Autodesk Fusion 360 part; units mm, degrees
(part 11 of 40)
  line L4767 (177.1415, 206.1712) -> (177.0096, 206.2642) construction
  line L4768 (177.0096, 206.2642) -> (176.8768, 206.3564) construction
  line L4769 (176.8768, 206.3564) -> (176.7434, 206.448) construction
  line L4770 (176.7434, 206.448) -> (176.6092, 206.5388) construction
  line L4771 (176.6092, 206.5388) -> (176.4743, 206.629) construction
  line L4772 (176.4743, 206.629) -> (176.3387, 206.7185) construction
  line L4773 (176.3387, 206.7185) -> (176.2025, 206.8073) construction
  line L4774 (176.2025, 206.8073) -> (176.0655, 206.8955) construction
  line L4775 (176.0655, 206.8955) -> (175.9278, 206.9829) construction
  line L4776 (175.9278, 206.9829) -> (175.7895, 207.0697) construction
  line L4777 (175.7895, 207.0697) -> (175.6505, 207.1558) construction
  line L4778 (175.6505, 207.1558) -> (175.5109, 207.2413) construction
  line L4779 (175.5109, 207.2413) -> (175.3706, 207.3261) construction
  line L4780 (175.3706, 207.3261) -> (175.2297, 207.4102) construction
  line L4781 (175.2297, 207.4102) -> (175.0882, 207.4937) construction
  line L4782 (175.0882, 207.4937) -> (174.946, 207.5765) construction
  line L4783 (174.946, 207.5765) -> (174.8032, 207.6587) construction
  line L4784 (174.8032, 207.6587) -> (174.6599, 207.7403) construction
  line L4785 (174.6599, 207.7403) -> (174.5159, 207.8212) construction
  line L4786 (174.5159, 207.8212) -> (174.3713, 207.9014) construction
  line L4787 (174.3713, 207.9014) -> (174.2262, 207.981) construction
  line L4788 (174.2262, 207.981) -> (174.0805, 208.06) construction
  line L4789 (174.0805, 208.06) -> (173.9342, 208.1383) construction
  line L4790 (173.9342, 208.1383) -> (173.7873, 208.216) construction
  line L4791 (173.7873, 208.216) -> (173.6399, 208.2931) construction
  line L4792 (173.6399, 208.2931) -> (173.4919, 208.3695) construction
  line L4793 (173.4919, 208.3695) -> (173.3434, 208.4453) construction
  line L4794 (173.3434, 208.4453) -> (173.1943, 208.5205) construction
  line L4795 (173.1943, 208.5205) -> (173.0447, 208.595) construction
  line L4796 (173.0447, 208.595) -> (172.8946, 208.669) construction
  line L4797 (172.8946, 208.669) -> (172.7439, 208.7423) construction
  line L4798 (172.7439, 208.7423) -> (172.5927, 208.8149) construction
  line L4799 (172.5927, 208.8149) -> (172.4411, 208.887) construction
  line L4800 (172.4411, 208.887) -> (172.2889, 208.9584) construction
  line L4801 (172.2889, 208.9584) -> (172.1667, 209.0151) construction
  line L4802 (172.1667, 209.0151) -> (172.0748, 209.0573) construction
  line L4803 (172.0748, 209.0573) -> (172.0135, 209.0853) construction
  line L4804 (172.0135, 209.0853) -> (171.9828, 209.0993) construction
  arc A128 (279.3511, 125.7868) -> (280.7456, 130.0785) centre (212.132, 150) ccw
  arc A129 (171.9828, 209.0993) -> (168.332, 206.4469) centre (212.132, 150) ccw
  spline S64 degree 5 poles (217.8271, 210.7685) (217.8299, 210.7993) (217.8349, 210.8609) (217.8398, 210.9533) (217.8417, 211.0766) (217.8376, 211.231) (217.8289, 211.3856) (217.8174, 211.5403) (217.8043, 211.695) (217.7903, 211.8498) (217.7751, 212.0045) (217.7585, 212.1593) (217.74, 212.314) (217.7191, 212.4688) (217.6961, 212.6235) (217.671, 212.7782) (217.6441, 212.9329) (217.6158, 213.0875) (217.5862, 213.2421) (217.5553, 213.3966) (217.5233, 213.5511) (217.4899, 213.7055) (217.4552, 213.8598) (217.4191, 214.014) (217.3817, 214.1682) (217.3429, 214.3222) (217.3029, 214.4762) (217.2617, 214.6301) (217.2193, 214.7839) (217.1759, 214.9376) (217.1313, 215.0912) (217.0856, 215.2447) (217.0388, 215.398) (216.9909, 215.5513) (216.9419, 215.7044) (216.8919, 215.8574) (216.8407, 216.0103) (216.7886, 216.1631) (216.7355, 216.3158) (216.6813, 216.4683) (216.6262, 216.6206) (216.57, 216.7729) (216.513, 216.925) (216.4549, 217.077) (216.3959, 217.2288) (216.3359, 217.3804) (216.275, 217.532) (216.2132, 217.6833) (216.1505, 217.8345) (216.0868, 217.9856) (216.0223, 218.1365) (215.9569, 218.2872) (215.8905, 218.4378) (215.8233, 218.5882) (215.7553, 218.7384) (215.6863, 218.8885) (215.6166, 219.0384) (215.5459, 219.1881) (215.4745, 219.3376) (215.4021, 219.487) (215.329, 219.6362) (215.255, 219.7852) (215.1802, 219.934) (215.1046, 220.0826) (215.0282, 220.2311) (214.951, 220.3793) (214.873, 220.5274) (214.7942, 220.6752) (214.7146, 220.8229) (214.6343, 220.9703) (214.5531, 221.1176) (214.4876, 221.2352) (214.4381, 221.3234) (214.4049, 221.3821) (214.3883, 221.4115) knots 0 0 0 0 0 0 0.01428571 0.02857143 0.04285714 0.05714286 0.07142857 0.08571429 0.1 0.11428571 0.12857143 0.14285714 0.15714286 0.17142857 0.18571429 0.2 0.21428571 0.22857143 0.24285714 0.25714286 0.27142857 0.28571429 0.3 0.31428571 0.32857143 0.34285714 0.35714286 0.37142857 0.38571429 0.4 0.41428571 0.42857143 0.44285714 0.45714286 0.47142857 0.48571429 0.5 0.51428571 0.52857143 0.54285714 0.55714286 0.57142857 0.58571429 0.6 0.61428571 0.62857143 0.64285714 0.65714286 0.67142857 0.68571429 0.7 0.71428571 0.72857143 0.74285714 0.75714286 0.77142857 0.78571429 0.8 0.81428571 0.82857143 0.84285714 0.85714286 0.87142857 0.88571429 0.9 0.91428571 0.92857143 0.94285714 0.95714286 0.97142857 0.98571429 1 1 1 1 1 1
  line L4805 (217.8271, 210.7685) -> (217.8299, 210.7993) construction
  line L4806 (217.8299, 210.7993) -> (217.8349, 210.8609) construction
  line L4807 (217.8349, 210.8609) -> (217.8398, 210.9533) construction
  line L4808 (217.8398, 210.9533) -> (217.8417, 211.0766) construction
  line L4809 (217.8417, 211.0766) -> (217.8376, 211.231) construction
  line L4810 (217.8376, 211.231) -> (217.8289, 211.3856) construction
  line L4811 (217.8289, 211.3856) -> (217.8174, 211.5403) construction
  line L4812 (217.8174, 211.5403) -> (217.8043, 211.695) construction
  line L4813 (217.8043, 211.695) -> (217.7903, 211.8498) construction
  line L4814 (217.7903, 211.8498) -> (217.7751, 212.0045) construction
  line L4815 (217.7751, 212.0045) -> (217.7585, 212.1593) construction
  line L4816 (217.7585, 212.1593) -> (217.74, 212.314) construction
  line L4817 (217.74, 212.314) -> (217.7191, 212.4688) construction
  line L4818 (217.7191, 212.4688) -> (217.6961, 212.6235) construction
  line L4819 (217.6961, 212.6235) -> (217.671, 212.7782) construction
  line L4820 (217.671, 212.7782) -> (217.6441, 212.9329) construction
  line L4821 (217.6441, 212.9329) -> (217.6158, 213.0875) construction
  line L4822 (217.6158, 213.0875) -> (217.5862, 213.2421) construction
  line L4823 (217.5862, 213.2421) -> (217.5553, 213.3966) construction
  line L4824 (217.5553, 213.3966) -> (217.5233, 213.5511) construction
  line L4825 (217.5233, 213.5511) -> (217.4899, 213.7055) construction
  line L4826 (217.4899, 213.7055) -> (217.4552, 213.8598) construction
  line L4827 (217.4552, 213.8598) -> (217.4191, 214.014) construction
  line L4828 (217.4191, 214.014) -> (217.3817, 214.1682) construction
  line L4829 (217.3817, 214.1682) -> (217.3429, 214.3222) construction
  line L4830 (217.3429, 214.3222) -> (217.3029, 214.4762) construction
  line L4831 (217.3029, 214.4762) -> (217.2617, 214.6301) construction
  line L4832 (217.2617, 214.6301) -> (217.2193, 214.7839) construction
  line L4833 (217.2193, 214.7839) -> (217.1759, 214.9376) construction
  line L4834 (217.1759, 214.9376) -> (217.1313, 215.0912) construction
  line L4835 (217.1313, 215.0912) -> (217.0856, 215.2447) construction
  line L4836 (217.0856, 215.2447) -> (217.0388, 215.398) construction
  line L4837 (217.0388, 215.398) -> (216.9909, 215.5513) construction
  line L4838 (216.9909, 215.5513) -> (216.9419, 215.7044) construction
  line L4839 (216.9419, 215.7044) -> (216.8919, 215.8574) construction
  line L4840 (216.8919, 215.8574) -> (216.8407, 216.0103) construction
  line L4841 (216.8407, 216.0103) -> (216.7886, 216.1631) construction
  line L4842 (216.7886, 216.1631) -> (216.7355, 216.3158) construction
  line L4843 (216.7355, 216.3158) -> (216.6813, 216.4683) construction
  line L4844 (216.6813, 216.4683) -> (216.6262, 216.6206) construction
  line L4845 (216.6262, 216.6206) -> (216.57, 216.7729) construction
  line L4846 (216.57, 216.7729) -> (216.513, 216.925) construction
  line L4847 (216.513, 216.925) -> (216.4549, 217.077) construction
  line L4848 (216.4549, 217.077) -> (216.3959, 217.2288) construction
  line L4849 (216.3959, 217.2288) -> (216.3359, 217.3804) construction
  line L4850 (216.3359, 217.3804) -> (216.275, 217.532) construction
  line L4851 (216.275, 217.532) -> (216.2132, 217.6833) construction
  line L4852 (216.2132, 217.6833) -> (216.1505, 217.8345) construction
  line L4853 (216.1505, 217.8345) -> (216.0868, 217.9856) construction
  line L4854 (216.0868, 217.9856) -> (216.0223, 218.1365) construction
  line L4855 (216.0223, 218.1365) -> (215.9569, 218.2872) construction
  line L4856 (215.9569, 218.2872) -> (215.8905, 218.4378) construction
  line L4857 (215.8905, 218.4378) -> (215.8233, 218.5882) construction
  line L4858 (215.8233, 218.5882) -> (215.7553, 218.7384) construction
  line L4859 (215.7553, 218.7384) -> (215.6863, 218.8885) construction
  line L4860 (215.6863, 218.8885) -> (215.6166, 219.0384) construction
  line L4861 (215.6166, 219.0384) -> (215.5459, 219.1881) construction
  line L4862 (215.5459, 219.1881) -> (215.4745, 219.3376) construction
  line L4863 (215.4745, 219.3376) -> (215.4021, 219.487) construction
  line L4864 (215.4021, 219.487) -> (215.329, 219.6362) construction
  line L4865 (215.329, 219.6362) -> (215.255, 219.7852) construction
  line L4866 (215.255, 219.7852) -> (215.1802, 219.934) construction
  line L4867 (215.1802, 219.934) -> (215.1046, 220.0826) construction
  line L4868 (215.1046, 220.0826) -> (215.0282, 220.2311) construction
  line L4869 (215.0282, 220.2311) -> (214.951, 220.3793) construction
  line L4870 (214.951, 220.3793) -> (214.873, 220.5274) construction
  line L4871 (214.873, 220.5274) -> (214.7942, 220.6752) construction
  line L4872 (214.7942, 220.6752) -> (214.7146, 220.8229) construction
  line L4873 (214.7146, 220.8229) -> (214.6343, 220.9703) construction
  line L4874 (214.6343, 220.9703) -> (214.5531, 221.1176) construction
  line L4875 (214.5531, 221.1176) -> (214.4876, 221.2352) construction
  line L4876 (214.4876, 221.2352) -> (214.4381, 221.3234) construction
  line L4877 (214.4381, 221.3234) -> (214.4049, 221.3821) construction
  line L4878 (214.4049, 221.3821) -> (214.3883, 221.4115) construction
  arc A130 (171.9828, 209.0993) -> (168.332, 206.4469) centre (212.132, 150) ccw
  spline S65 degree 5 poles (217.8271, 210.7685) (217.8299, 210.7993) (217.8349, 210.8609) (217.8398, 210.9533) (217.8417, 211.0766) (217.8376, 211.231) (217.8289, 211.3856) (217.8174, 211.5403) (217.8043, 211.695) (217.7903, 211.8498) (217.7751, 212.0045) (217.7585, 212.1593) (217.74, 212.314) (217.7191, 212.4688) (217.6961, 212.6235) (217.671, 212.7782) (217.6441, 212.9329) (217.6158, 213.0875) (217.5862, 213.2421) (217.5553, 213.3966) (217.5233, 213.5511) (217.4899, 213.7055) (217.4552, 213.8598) (217.4191, 214.014) (217.3817, 214.1682) (217.3429, 214.3222) (217.3029, 214.4762) (217.2617, 214.6301) (217.2193, 214.7839) (217.1759, 214.9376) (217.1313, 215.0912) (217.0856, 215.2447) (217.0388, 215.398) (216.9909, 215.5513) (216.9419, 215.7044) (216.8919, 215.8574) (216.8407, 216.0103) (216.7886, 216.1631) (216.7355, 216.3158) (216.6813, 216.4683) (216.6262, 216.6206) (216.57, 216.7729) (216.513, 216.925) (216.4549, 217.077) (216.3959, 217.2288) (216.3359, 217.3804) (216.275, 217.532) (216.2132, 217.6833) (216.1505, 217.8345) (216.0868, 217.9856) (216.0223, 218.1365) (215.9569, 218.2872) (215.8905, 218.4378) (215.8233, 218.5882) (215.7553, 218.7384) (215.6863, 218.8885) (215.6166, 219.0384) (215.5459, 219.1881) (215.4745, 219.3376) (215.4021, 219.487) (215.329, 219.6362) (215.255, 219.7852) (215.1802, 219.934) (215.1046, 220.0826) (215.0282, 220.2311) (214.951, 220.3793) (214.873, 220.5274) (214.7942, 220.6752) (214.7146, 220.8229) (214.6343, 220.9703) (214.5531, 221.1176) (214.4876, 221.2352) (214.4381, 221.3234) (214.4049, 221.3821) (214.3883, 221.4115) knots 0 0 0 0 0 0 0.01428571 0.02857143 0.04285714 0.05714286 0.07142857 0.08571429 0.1 0.11428571 0.12857143 0.14285714 0.15714286 0.17142857 0.18571429 0.2 0.21428571 0.22857143 0.24285714 0.25714286 0.27142857 0.28571429 0.3 0.31428571 0.32857143 0.34285714 0.35714286 0.37142857 0.38571429 0.4 0.41428571 0.42857143 0.44285714 0.45714286 0.47142857 0.48571429 0.5 0.51428571 0.52857143 0.54285714 0.55714286 0.57142857 0.58571429 0.6 0.61428571 0.62857143 0.64285714 0.65714286 0.67142857 0.68571429 0.7 0.71428571 0.72857143 0.74285714 0.75714286 0.77142857 0.78571429 0.8 0.81428571 0.82857143 0.84285714 0.85714286 0.87142857 0.88571429 0.9 0.91428571 0.92857143 0.94285714 0.95714286 0.97142857 0.98571429 1 1 1 1 1 1
  line L4879 (217.8271, 210.7685) -> (217.8299, 210.7993) construction
  line L4880 (217.8299, 210.7993) -> (217.8349, 210.8609) construction
  line L4881 (217.8349, 210.8609) -> (217.8398, 210.9533) construction
  line L4882 (217.8398, 210.9533) -> (217.8417, 211.0766) construction
  line L4883 (217.8417, 211.0766) -> (217.8376, 211.231) construction
  line L4884 (217.8376, 211.231) -> (217.8289, 211.3856) construction
  line L4885 (217.8289, 211.3856) -> (217.8174, 211.5403) construction
  line L4886 (217.8174, 211.5403) -> (217.8043, 211.695) construction
  line L4887 (217.8043, 211.695) -> (217.7903, 211.8498) construction
  line L4888 (217.7903, 211.8498) -> (217.7751, 212.0045) construction
  line L4889 (217.7751, 212.0045) -> (217.7585, 212.1593) construction
  line L4890 (217.7585, 212.1593) -> (217.74, 212.314) construction
  line L4891 (217.74, 212.314) -> (217.7191, 212.4688) construction
  line L4892 (217.7191, 212.4688) -> (217.6961, 212.6235) construction
  line L4893 (217.6961, 212.6235) -> (217.671, 212.7782) construction
  line L4894 (217.671, 212.7782) -> (217.6441, 212.9329) construction
  line L4895 (217.6441, 212.9329) -> (217.6158, 213.0875) construction
  line L4896 (217.6158, 213.0875) -> (217.5862, 213.2421) construction
  line L4897 (217.5862, 213.2421) -> (217.5553, 213.3966) construction
  line L4898 (217.5553, 213.3966) -> (217.5233, 213.5511) construction
  line L4899 (217.5233, 213.5511) -> (217.4899, 213.7055) construction
  line L4900 (217.4899, 213.7055) -> (217.4552, 213.8598) construction
  line L4901 (217.4552, 213.8598) -> (217.4191, 214.014) construction
  line L4902 (217.4191, 214.014) -> (217.3817, 214.1682) construction
  line L4903 (217.3817, 214.1682) -> (217.3429, 214.3222) construction
  line L4904 (217.3429, 214.3222) -> (217.3029, 214.4762) construction
  line L4905 (217.3029, 214.4762) -> (217.2617, 214.6301) construction
  line L4906 (217.2617, 214.6301) -> (217.2193, 214.7839) construction
  line L4907 (217.2193, 214.7839) -> (217.1759, 214.9376) construction
  line L4908 (217.1759, 214.9376) -> (217.1313, 215.0912) construction
  line L4909 (217.1313, 215.0912) -> (217.0856, 215.2447) construction
  line L4910 (217.0856, 215.2447) -> (217.0388, 215.398) construction
  line L4911 (217.0388, 215.398) -> (216.9909, 215.5513) construction
  line L4912 (216.9909, 215.5513) -> (216.9419, 215.7044) construction
  line L4913 (216.9419, 215.7044) -> (216.8919, 215.8574) construction
  line L4914 (216.8919, 215.8574) -> (216.8407, 216.0103) construction
  line L4915 (216.8407, 216.0103) -> (216.7886, 216.1631) construction
  line L4916 (216.7886, 216.1631) -> (216.7355, 216.3158) construction
  line L4917 (216.7355, 216.3158) -> (216.6813, 216.4683) construction
  line L4918 (216.6813, 216.4683) -> (216.6262, 216.6206) construction
  line L4919 (216.6262, 216.6206) -> (216.57, 216.7729) construction
  line L4920 (216.57, 216.7729) -> (216.513, 216.925) construction
  line L4921 (216.513, 216.925) -> (216.4549, 217.077) construction
  line L4922 (216.4549, 217.077) -> (216.3959, 217.2288) construction
  line L4923 (216.3959, 217.2288) -> (216.3359, 217.3804) construction
  line L4924 (216.3359, 217.3804) -> (216.275, 217.532) construction
  line L4925 (216.275, 217.532) -> (216.2132, 217.6833) construction
  line L4926 (216.2132, 217.6833) -> (216.1505, 217.8345) construction
  line L4927 (216.1505, 217.8345) -> (216.0868, 217.9856) construction
  line L4928 (216.0868, 217.9856) -> (216.0223, 218.1365) construction
  line L4929 (216.0223, 218.1365) -> (215.9569, 218.2872) construction
  line L4930 (215.9569, 218.2872) -> (215.8905, 218.4378) construction
  line L4931 (215.8905, 218.4378) -> (215.8233, 218.5882) construction
  line L4932 (215.8233, 218.5882) -> (215.7553, 218.7384) construction
  line L4933 (215.7553, 218.7384) -> (215.6863, 218.8885) construction
  line L4934 (215.6863, 218.8885) -> (215.6166, 219.0384) construction
  line L4935 (215.6166, 219.0384) -> (215.5459, 219.1881) construction
  line L4936 (215.5459, 219.1881) -> (215.4745, 219.3376) construction
  line L4937 (215.4745, 219.3376) -> (215.4021, 219.487) construction
  line L4938 (215.4021, 219.487) -> (215.329, 219.6362) construction
  line L4939 (215.329, 219.6362) -> (215.255, 219.7852) construction
  line L4940 (215.255, 219.7852) -> (215.1802, 219.934) construction
  line L4941 (215.1802, 219.934) -> (215.1046, 220.0826) construction
  line L4942 (215.1046, 220.0826) -> (215.0282, 220.2311) construction
  line L4943 (215.0282, 220.2311) -> (214.951, 220.3793) construction
  line L4944 (214.951, 220.3793) -> (214.873, 220.5274) construction
  line L4945 (214.873, 220.5274) -> (214.7942, 220.6752) construction
  line L4946 (214.7942, 220.6752) -> (214.7146, 220.8229) construction
  line L4947 (214.7146, 220.8229) -> (214.6343, 220.9703) construction
  line L4948 (214.6343, 220.9703) -> (214.5531, 221.1176) construction
  line L4949 (214.5531, 221.1176) -> (214.4876, 221.2352) construction
  line L4950 (214.4876, 221.2352) -> (214.4381, 221.3234) construction
  line L4951 (214.4381, 221.3234) -> (214.4049, 221.3821) construction
  line L4952 (214.4049, 221.3821) -> (214.3883, 221.4115) construction
  spline S66 degree 5 poles (206.4369, 210.7685) (206.4341, 210.7993) (206.4291, 210.8609) (206.4242, 210.9533) (206.4223, 211.0766) (206.4264, 211.231) (206.4351, 211.3856) (206.4466, 211.5403) (206.4597, 211.695) (206.4737, 211.8498) (206.4889, 212.0045) (206.5055, 212.1593) (206.524, 212.314) (206.5449, 212.4688) (206.5679, 212.6235) (206.593, 212.7782) (206.6199, 212.9329) (206.6482, 213.0875) (206.6778, 213.2421) (206.7087, 213.3966) (206.7407, 213.5511) (206.7741, 213.7055) (206.8088, 213.8598) (206.8449, 214.014) (206.8823, 214.1682) (206.9211, 214.3222) (206.9611, 214.4762) (207.0023, 214.6301) (207.0447, 214.7839) (207.0881, 214.9376) (207.1327, 215.0912) (207.1784, 215.2447) (207.2252, 215.398) (207.2731, 215.5513) (207.3221, 215.7044) (207.3721, 215.8574) (207.4233, 216.0103) (207.4754, 216.1631) (207.5285, 216.3158) (207.5827, 216.4683) (207.6378, 216.6206) (207.694, 216.7729) (207.751, 216.925) (207.8091, 217.077) (207.8681, 217.2288) (207.9281, 217.3804) (207.989, 217.532) (208.0508, 217.6833) (208.1135, 217.8345) (208.1772, 217.9856) (208.2417, 218.1365) (208.3071, 218.2872) (208.3735, 218.4378) (208.4407, 218.5882) (208.5087, 218.7384) (208.5777, 218.8885) (208.6474, 219.0384) (208.7181, 219.1881) (208.7895, 219.3376) (208.8619, 219.487) (208.935, 219.6362) (209.009, 219.7852) (209.0838, 219.934) (209.1594, 220.0826) (209.2358, 220.2311) (209.313, 220.3793) (209.391, 220.5274) (209.4698, 220.6752) (209.5494, 220.8229) (209.6297, 220.9703) (209.7109, 221.1176) (209.7764, 221.2352) (209.8259, 221.3234) (209.8591, 221.3821) (209.8757, 221.4115) knots 0 0 0 0 0 0 0.01428571 0.02857143 0.04285714 0.05714286 0.07142857 0.08571429 0.1 0.11428571 0.12857143 0.14285714 0.15714286 0.17142857 0.18571429 0.2 0.21428571 0.22857143 0.24285714 0.25714286 0.27142857 0.28571429 0.3 0.31428571 0.32857143 0.34285714 0.35714286 0.37142857 0.38571429 0.4 0.41428571 0.42857143 0.44285714 0.45714286 0.47142857 0.48571429 0.5 0.51428571 0.52857143 0.54285714 0.55714286 0.57142857 0.58571429 0.6 0.61428571 0.62857143 0.64285714 0.65714286 0.67142857 0.68571429 0.7 0.71428571 0.72857143 0.74285714 0.75714286 0.77142857 0.78571429 0.8 0.81428571 0.82857143 0.84285714 0.85714286 0.87142857 0.88571429 0.9 0.91428571 0.92857143 0.94285714 0.95714286 0.97142857 0.98571429 1 1 1 1 1 1
  line L4953 (206.4369, 210.7685) -> (206.4341, 210.7993) construction
  line L4954 (206.4341, 210.7993) -> (206.4291, 210.8609) construction
  line L4955 (206.4291, 210.8609) -> (206.4242, 210.9533) construction
  line L4956 (206.4242, 210.9533) -> (206.4223, 211.0766) construction
  line L4957 (206.4223, 211.0766) -> (206.4264, 211.231) construction
  line L4958 (206.4264, 211.231) -> (206.4351, 211.3856) construction
  line L4959 (206.4351, 211.3856) -> (206.4466, 211.5403) construction
  line L4960 (206.4466, 211.5403) -> (206.4597, 211.695) construction
  line L4961 (206.4597, 211.695) -> (206.4737, 211.8498) construction
  line L4962 (206.4737, 211.8498) -> (206.4889, 212.0045) construction
  line L4963 (206.4889, 212.0045) -> (206.5055, 212.1593) construction
  line L4964 (206.5055, 212.1593) -> (206.524, 212.314) construction
  line L4965 (206.524, 212.314) -> (206.5449, 212.4688) construction
  line L4966 (206.5449, 212.4688) -> (206.5679, 212.6235) construction
  line L4967 (206.5679, 212.6235) -> (206.593, 212.7782) construction
  line L4968 (206.593, 212.7782) -> (206.6199, 212.9329) construction
  line L4969 (206.6199, 212.9329) -> (206.6482, 213.0875) construction
  line L4970 (206.6482, 213.0875) -> (206.6778, 213.2421) construction
  line L4971 (206.6778, 213.2421) -> (206.7087, 213.3966) construction
  line L4972 (206.7087, 213.3966) -> (206.7407, 213.5511) construction
  line L4973 (206.7407, 213.5511) -> (206.7741, 213.7055) construction
  line L4974 (206.7741, 213.7055) -> (206.8088, 213.8598) construction
  line L4975 (206.8088, 213.8598) -> (206.8449, 214.014) construction
  line L4976 (206.8449, 214.014) -> (206.8823, 214.1682) construction
  line L4977 (206.8823, 214.1682) -> (206.9211, 214.3222) construction
  line L4978 (206.9211, 214.3222) -> (206.9611, 214.4762) construction
  line L4979 (206.9611, 214.4762) -> (207.0023, 214.6301) construction
  line L4980 (207.0023, 214.6301) -> (207.0447, 214.7839) construction
  line L4981 (207.0447, 214.7839) -> (207.0881, 214.9376) construction
  line L4982 (207.0881, 214.9376) -> (207.1327, 215.0912) construction
  line L4983 (207.1327, 215.0912) -> (207.1784, 215.2447) construction
  line L4984 (207.1784, 215.2447) -> (207.2252, 215.398) construction
  line L4985 (207.2252, 215.398) -> (207.2731, 215.5513) construction
  line L4986 (207.2731, 215.5513) -> (207.3221, 215.7044) construction
  line L4987 (207.3221, 215.7044) -> (207.3721, 215.8574) construction
  line L4988 (207.3721, 215.8574) -> (207.4233, 216.0103) construction
  line L4989 (207.4233, 216.0103) -> (207.4754, 216.1631) construction
  line L4990 (207.4754, 216.1631) -> (207.5285, 216.3158) construction
  line L4991 (207.5285, 216.3158) -> (207.5827, 216.4683) construction
  line L4992 (207.5827, 216.4683) -> (207.6378, 216.6206) construction
  line L4993 (207.6378, 216.6206) -> (207.694, 216.7729) construction
  line L4994 (207.694, 216.7729) -> (207.751, 216.925) construction
  line L4995 (207.751, 216.925) -> (207.8091, 217.077) construction
  line L4996 (207.8091, 217.077) -> (207.8681, 217.2288) construction
  line L4997 (207.8681, 217.2288) -> (207.9281, 217.3804) construction
  line L4998 (207.9281, 217.3804) -> (207.989, 217.532) construction
  line L4999 (207.989, 217.532) -> (208.0508, 217.6833) construction
  line L5000 (208.0508, 217.6833) -> (208.1135, 217.8345) construction
  line L5001 (208.1135, 217.8345) -> (208.1772, 217.9856) construction
  line L5002 (208.1772, 217.9856) -> (208.2417, 218.1365) construction
  line L5003 (208.2417, 218.1365) -> (208.3071, 218.2872) construction
  line L5004 (208.3071, 218.2872) -> (208.3735, 218.4378) construction
  line L5005 (208.3735, 218.4378) -> (208.4407, 218.5882) construction
  line L5006 (208.4407, 218.5882) -> (208.5087, 218.7384) construction
  line L5007 (208.5087, 218.7384) -> (208.5777, 218.8885) construction
  line L5008 (208.5777, 218.8885) -> (208.6474, 219.0384) construction
  line L5009 (208.6474, 219.0384) -> (208.7181, 219.1881) construction
  line L5010 (208.7181, 219.1881) -> (208.7895, 219.3376) construction
  line L5011 (208.7895, 219.3376) -> (208.8619, 219.487) construction
  line L5012 (208.8619, 219.487) -> (208.935, 219.6362) construction
  line L5013 (208.935, 219.6362) -> (209.009, 219.7852) construction
  line L5014 (209.009, 219.7852) -> (209.0838, 219.934) construction
  line L5015 (209.0838, 219.934) -> (209.1594, 220.0826) construction
  line L5016 (209.1594, 220.0826) -> (209.2358, 220.2311) construction
  line L5017 (209.2358, 220.2311) -> (209.313, 220.3793) construction
  line L5018 (209.313, 220.3793) -> (209.391, 220.5274) construction
  line L5019 (209.391, 220.5274) -> (209.4698, 220.6752) construction
  line L5020 (209.4698, 220.6752) -> (209.5494, 220.8229) construction
  line L5021 (209.5494, 220.8229) -> (209.6297, 220.9703) construction
  line L5022 (209.6297, 220.9703) -> (209.7109, 221.1176) construction
  line L5023 (209.7109, 221.1176) -> (209.7764, 221.2352) construction
  line L5024 (209.7764, 221.2352) -> (209.8259, 221.3234) construction
  line L5025 (209.8259, 221.3234) -> (209.8591, 221.3821) construction
  line L5026 (209.8591, 221.3821) -> (209.8757, 221.4115) construction
  spline S67 degree 5 poles (206.4369, 210.7685) (206.4341, 210.7993) (206.4291, 210.8609) (206.4242, 210.9533) (206.4223, 211.0766) (206.4264, 211.231) (206.4351, 211.3856) (206.4466, 211.5403) (206.4597, 211.695) (206.4737, 211.8498) (206.4889, 212.0045) (206.5055, 212.1593) (206.524, 212.314) (206.5449, 212.4688) (206.5679, 212.6235) (206.593, 212.7782) (206.6199, 212.9329) (206.6482, 213.0875) (206.6778, 213.2421) (206.7087, 213.3966) (206.7407, 213.5511) (206.7741, 213.7055) (206.8088, 213.8598) (206.8449, 214.014) (206.8823, 214.1682) (206.9211, 214.3222) (206.9611, 214.4762) (207.0023, 214.6301) (207.0447, 214.7839) (207.0881, 214.9376) (207.1327, 215.0912) (207.1784, 215.2447) (207.2252, 215.398) (207.2731, 215.5513) (207.3221, 215.7044) (207.3721, 215.8574) (207.4233, 216.0103) (207.4754, 216.1631) (207.5285, 216.3158) (207.5827, 216.4683) (207.6378, 216.6206) (207.694, 216.7729) (207.751, 216.925) (207.8091, 217.077) (207.8681, 217.2288) (207.9281, 217.3804) (207.989, 217.532) (208.0508, 217.6833) (208.1135, 217.8345) (208.1772, 217.9856) (208.2417, 218.1365) (208.3071, 218.2872) (208.3735, 218.4378) (208.4407, 218.5882) (208.5087, 218.7384) (208.5777, 218.8885) (208.6474, 219.0384) (208.7181, 219.1881) (208.7895, 219.3376) (208.8619, 219.487) (208.935, 219.6362) (209.009, 219.7852) (209.0838, 219.934) (209.1594, 220.0826) (209.2358, 220.2311) (209.313, 220.3793) (209.391, 220.5274) (209.4698, 220.6752) (209.5494, 220.8229) (209.6297, 220.9703) (209.7109, 221.1176) (209.7764, 221.2352) (209.8259, 221.3234) (209.8591, 221.3821) (209.8757, 221.4115) knots 0 0 0 0 0 0 0.01428571 0.02857143 0.04285714 0.05714286 0.07142857 0.08571429 0.1 0.11428571 0.12857143 0.14285714 0.15714286 0.17142857 0.18571429 0.2 0.21428571 0.22857143 0.24285714 0.25714286 0.27142857 0.28571429 0.3 0.31428571 0.32857143 0.34285714 0.35714286 0.37142857 0.38571429 0.4 0.41428571 0.42857143 0.44285714 0.45714286 0.47142857 0.48571429 0.5 0.51428571 0.52857143 0.54285714 0.55714286 0.57142857 0.58571429 0.6 0.61428571 0.62857143 0.64285714 0.65714286 0.67142857 0.68571429 0.7 0.71428571 0.72857143 0.74285714 0.75714286 0.77142857 0.78571429 0.8 0.81428571 0.82857143 0.84285714 0.85714286 0.87142857 0.88571429 0.9 0.91428571 0.92857143 0.94285714 0.95714286 0.97142857 0.98571429 1 1 1 1 1 1
  line L5027 (206.4369, 210.7685) -> (206.4341, 210.7993) construction
  line L5028 (206.4341, 210.7993) -> (206.4291, 210.8609) construction
  line L5029 (206.4291, 210.8609) -> (206.4242, 210.9533) construction
  line L5030 (206.4242, 210.9533) -> (206.4223, 211.0766) construction
  line L5031 (206.4223, 211.0766) -> (206.4264, 211.231) construction
  line L5032 (206.4264, 211.231) -> (206.4351, 211.3856) construction
  line L5033 (206.4351, 211.3856) -> (206.4466, 211.5403) construction
  line L5034 (206.4466, 211.5403) -> (206.4597, 211.695) construction
  line L5035 (206.4597, 211.695) -> (206.4737, 211.8498) construction
  line L5036 (206.4737, 211.8498) -> (206.4889, 212.0045) construction
  line L5037 (206.4889, 212.0045) -> (206.5055, 212.1593) construction
  line L5038 (206.5055, 212.1593) -> (206.524, 212.314) construction
  line L5039 (206.524, 212.314) -> (206.5449, 212.4688) construction
  line L5040 (206.5449, 212.4688) -> (206.5679, 212.6235) construction
  line L5041 (206.5679, 212.6235) -> (206.593, 212.7782) construction
  line L5042 (206.593, 212.7782) -> (206.6199, 212.9329) construction
  line L5043 (206.6199, 212.9329) -> (206.6482, 213.0875) construction
  line L5044 (206.6482, 213.0875) -> (206.6778, 213.2421) construction
  line L5045 (206.6778, 213.2421) -> (206.7087, 213.3966) construction
  line L5046 (206.7087, 213.3966) -> (206.7407, 213.5511) construction
  line L5047 (206.7407, 213.5511) -> (206.7741, 213.7055) construction
  line L5048 (206.7741, 213.7055) -> (206.8088, 213.8598) construction
  line L5049 (206.8088, 213.8598) -> (206.8449, 214.014) construction
  line L5050 (206.8449, 214.014) -> (206.8823, 214.1682) construction
  line L5051 (206.8823, 214.1682) -> (206.9211, 214.3222) construction
  line L5052 (206.9211, 214.3222) -> (206.9611, 214.4762) construction
  line L5053 (206.9611, 214.4762) -> (207.0023, 214.6301) construction
  line L5054 (207.0023, 214.6301) -> (207.0447, 214.7839) construction
  line L5055 (207.0447, 214.7839) -> (207.0881, 214.9376) construction
  line L5056 (207.0881, 214.9376) -> (207.1327, 215.0912) construction
  line L5057 (207.1327, 215.0912) -> (207.1784, 215.2447) construction
  line L5058 (207.1784, 215.2447) -> (207.2252, 215.398) construction
  line L5059 (207.2252, 215.398) -> (207.2731, 215.5513) construction
  line L5060 (207.2731, 215.5513) -> (207.3221, 215.7044) construction
  line L5061 (207.3221, 215.7044) -> (207.3721, 215.8574) construction
  line L5062 (207.3721, 215.8574) -> (207.4233, 216.0103) construction
  line L5063 (207.4233, 216.0103) -> (207.4754, 216.1631) construction
  line L5064 (207.4754, 216.1631) -> (207.5285, 216.3158) construction
  line L5065 (207.5285, 216.3158) -> (207.5827, 216.4683) construction
  line L5066 (207.5827, 216.4683) -> (207.6378, 216.6206) construction
  line L5067 (207.6378, 216.6206) -> (207.694, 216.7729) construction
  line L5068 (207.694, 216.7729) -> (207.751, 216.925) construction
  line L5069 (207.751, 216.925) -> (207.8091, 217.077) construction
  line L5070 (207.8091, 217.077) -> (207.8681, 217.2288) construction
  line L5071 (207.8681, 217.2288) -> (207.9281, 217.3804) construction
  line L5072 (207.9281, 217.3804) -> (207.989, 217.532) construction
  line L5073 (207.989, 217.532) -> (208.0508, 217.6833) construction
  line L5074 (208.0508, 217.6833) -> (208.1135, 217.8345) construction
  line L5075 (208.1135, 217.8345) -> (208.1772, 217.9856) construction
  line L5076 (208.1772, 217.9856) -> (208.2417, 218.1365) construction
  line L5077 (208.2417, 218.1365) -> (208.3071, 218.2872) construction
  line L5078 (208.3071, 218.2872) -> (208.3735, 218.4378) construction
  line L5079 (208.3735, 218.4378) -> (208.4407, 218.5882) construction
  line L5080 (208.4407, 218.5882) -> (208.5087, 218.7384) construction
  line L5081 (208.5087, 218.7384) -> (208.5777, 218.8885) construction
  line L5082 (208.5777, 218.8885) -> (208.6474, 219.0384) construction
  line L5083 (208.6474, 219.0384) -> (208.7181, 219.1881) construction
  line L5084 (208.7181, 219.1881) -> (208.7895, 219.3376) construction
  line L5085 (208.7895, 219.3376) -> (208.8619, 219.487) construction
  line L5086 (208.8619, 219.487) -> (208.935, 219.6362) construction
  line L5087 (208.935, 219.6362) -> (209.009, 219.7852) construction
  line L5088 (209.009, 219.7852) -> (209.0838, 219.934) construction
  line L5089 (209.0838, 219.934) -> (209.1594, 220.0826) construction
  line L5090 (209.1594, 220.0826) -> (209.2358, 220.2311) construction
  line L5091 (209.2358, 220.2311) -> (209.313, 220.3793) construction
  line L5092 (209.313, 220.3793) -> (209.391, 220.5274) construction
  line L5093 (209.391, 220.5274) -> (209.4698, 220.6752) construction
  line L5094 (209.4698, 220.6752) -> (209.5494, 220.8229) construction
  line L5095 (209.5494, 220.8229) -> (209.6297, 220.9703) construction
  line L5096 (209.6297, 220.9703) -> (209.7109, 221.1176) construction
  line L5097 (209.7109, 221.1176) -> (209.7764, 221.2352) construction
  line L5098 (209.7764, 221.2352) -> (209.8259, 221.3234) construction
  line L5099 (209.8259, 221.3234) -> (209.8591, 221.3821) construction
  line L5100 (209.8591, 221.3821) -> (209.8757, 221.4115) construction
  arc A131 (204.8514, 206.9737) -> (206.5892, 209.1442) centre (204.5979, 208.9575) ccw
  arc A132 (204.8514, 206.9737) -> (206.5892, 209.1442) centre (204.5979, 208.9575) ccw
  arc A133 (204.8514, 206.9737) -> (201.4504, 206.435) centre (212.132, 150) ccw
  arc A134 (204.8514, 206.9737) -> (201.4504, 206.435) centre (212.132, 150) ccw
  line L5101 (206.5892, 209.1442) -> (206.4369, 210.7685)
  line L5102 (206.5892, 209.1442) -> (206.4369, 210.7685)
  arc A135 (217.6748, 209.1442) -> (219.4126, 206.9737) centre (219.6661, 208.9575) ccw
  arc A136 (217.6748, 209.1442) -> (219.4126, 206.9737) centre (219.6661, 208.9575) ccw
  line L5103 (217.6748, 209.1442) -> (217.8271, 210.7685)
  line L5104 (217.6748, 209.1442) -> (217.8271, 210.7685)
  line L5105 (161.0254, 119.7202) -> (159.6217, 118.8885)
  line L5106 (152.9878, 155.5428) -> (151.3635, 155.6951)
  spline S68 degree 5 poles (159.6217, 181.1115) (159.5952, 181.1272) (159.5425, 181.1594) (159.4648, 181.2097) (159.3639, 181.2807) (159.2414, 181.3748) (159.1214, 181.4727) (159.0031, 181.5729) (158.8856, 181.6744) (158.7686, 181.7767) (158.6523, 181.88) (158.5369, 181.9844) (158.4226, 182.0903) (158.3096, 182.1981) (158.198, 182.3077) (158.0876, 182.419) (157.9783, 182.5316) (157.8698, 182.6455) (157.7622, 182.7603) (157.6553, 182.876) (157.5492, 182.9927) (157.4439, 183.1105) (157.3394, 183.2292) (157.2359, 183.3491) (157.1332, 183.47) (157.0313, 183.5919) (156.9303, 183.7148) (156.83, 183.8386) (156.7305, 183.9633) (156.6317, 184.0888) (156.5336, 184.2151) (156.4363, 184.3423) (156.3397, 184.4703) (156.2439, 184.5991) (156.1488, 184.7288) (156.0544, 184.8592) (155.9608, 184.9905) (155.8678, 185.1224) (155.7756, 185.2552) (155.684, 185.3886) (155.5932, 185.5228) (155.503, 185.6577) (155.4135, 185.7933) (155.3247, 185.9295) (155.2365, 186.0665) (155.1491, 186.2042) (155.0623, 186.3425) (154.9762, 186.4815) (154.8907, 186.6211) (154.8059, 186.7614) (154.7218, 186.9023) (154.6383, 187.0438) (154.5555, 187.186) (154.4733, 187.3288) (154.3917, 187.4721) (154.3108, 187.6161) (154.2306, 187.7607) (154.151, 187.9058) (154.072, 188.0515) (153.9937, 188.1978) (153.916, 188.3447) (153.8389, 188.4921) (153.7625, 188.6401) (153.6867, 188.7886) (153.6115, 188.9377) (153.537, 189.0873) (153.463, 189.2374) (153.3897, 189.3881) (153.3171, 189.5393) (153.245, 189.6909) (153.1736, 189.8431) (153.1169, 189.9653) (153.0747, 190.0572) (153.0467, 190.1185) (153.0327, 190.1492) knots 0 0 0 0 0 0 0.01428571 0.02857143 0.04285714 0.05714286 0.07142857 0.08571429 0.1 0.11428571 0.12857143 0.14285714 0.15714286 0.17142857 0.18571429 0.2 0.21428571 0.22857143 0.24285714 0.25714286 0.27142857 0.28571429 0.3 0.31428571 0.32857143 0.34285714 0.35714286 0.37142857 0.38571429 0.4 0.41428571 0.42857143 0.44285714 0.45714286 0.47142857 0.48571429 0.5 0.51428571 0.52857143 0.54285714 0.55714286 0.57142857 0.58571429 0.6 0.61428571 0.62857143 0.64285714 0.65714286 0.67142857 0.68571429 0.7 0.71428571 0.72857143 0.74285714 0.75714286 0.77142857 0.78571429 0.8 0.81428571 0.82857143 0.84285714 0.85714286 0.87142857 0.88571429 0.9 0.91428571 0.92857143 0.94285714 0.95714286 0.97142857 0.98571429 1 1 1 1 1 1
  line L5107 (159.6217, 181.1115) -> (159.5952, 181.1272) construction
  line L5108 (159.5952, 181.1272) -> (159.5425, 181.1594) construction
  line L5109 (159.5425, 181.1594) -> (159.4648, 181.2097) construction
  line L5110 (159.4648, 181.2097) -> (159.3639, 181.2807) construction
  line L5111 (159.3639, 181.2807) -> (159.2414, 181.3748) construction
  line L5112 (159.2414, 181.3748) -> (159.1214, 181.4727) construction
  line L5113 (159.1214, 181.4727) -> (159.0031, 181.5729) construction
  line L5114 (159.0031, 181.5729) -> (158.8856, 181.6744) construction
  line L5115 (158.8856, 181.6744) -> (158.7686, 181.7767) construction
  line L5116 (158.7686, 181.7767) -> (158.6523, 181.88) construction
  line L5117 (158.6523, 181.88) -> (158.5369, 181.9844) construction
  line L5118 (158.5369, 181.9844) -> (158.4226, 182.0903) construction
  line L5119 (158.4226, 182.0903) -> (158.3096, 182.1981) construction
  line L5120 (158.3096, 182.1981) -> (158.198, 182.3077) construction
  line L5121 (158.198, 182.3077) -> (158.0876, 182.419) construction
  line L5122 (158.0876, 182.419) -> (157.9783, 182.5316) construction
  line L5123 (157.9783, 182.5316) -> (157.8698, 182.6455) construction
  line L5124 (157.8698, 182.6455) -> (157.7622, 182.7603) construction
  line L5125 (157.7622, 182.7603) -> (157.6553, 182.876) construction
  line L5126 (157.6553, 182.876) -> (157.5492, 182.9927) construction
  line L5127 (157.5492, 182.9927) -> (157.4439, 183.1105) construction
  line L5128 (157.4439, 183.1105) -> (157.3394, 183.2292) construction
  line L5129 (157.3394, 183.2292) -> (157.2359, 183.3491) construction
  line L5130 (157.2359, 183.3491) -> (157.1332, 183.47) construction
  line L5131 (157.1332, 183.47) -> (157.0313, 183.5919) construction
  line L5132 (157.0313, 183.5919) -> (156.9303, 183.7148) construction
  line L5133 (156.9303, 183.7148) -> (156.83, 183.8386) construction
  line L5134 (156.83, 183.8386) -> (156.7305, 183.9633) construction
  line L5135 (156.7305, 183.9633) -> (156.6317, 184.0888) construction
  line L5136 (156.6317, 184.0888) -> (156.5336, 184.2151) construction
  line L5137 (156.5336, 184.2151) -> (156.4363, 184.3423) construction
  line L5138 (156.4363, 184.3423) -> (156.3397, 184.4703) construction
  line L5139 (156.3397, 184.4703) -> (156.2439, 184.5991) construction
  line L5140 (156.2439, 184.5991) -> (156.1488, 184.7288) construction
  line L5141 (156.1488, 184.7288) -> (156.0544, 184.8592) construction
  line L5142 (156.0544, 184.8592) -> (155.9608, 184.9905) construction
  line L5143 (155.9608, 184.9905) -> (155.8678, 185.1224) construction
  line L5144 (155.8678, 185.1224) -> (155.7756, 185.2552) construction
  line L5145 (155.7756, 185.2552) -> (155.684, 185.3886) construction
  line L5146 (155.684, 185.3886) -> (155.5932, 185.5228) construction
  line L5147 (155.5932, 185.5228) -> (155.503, 185.6577) construction
  line L5148 (155.503, 185.6577) -> (155.4135, 185.7933) construction
  line L5149 (155.4135, 185.7933) -> (155.3247, 185.9295) construction
  line L5150 (155.3247, 185.9295) -> (155.2365, 186.0665) construction
  line L5151 (155.2365, 186.0665) -> (155.1491, 186.2042) construction
  line L5152 (155.1491, 186.2042) -> (155.0623, 186.3425) construction
  line L5153 (155.0623, 186.3425) -> (154.9762, 186.4815) construction
  line L5154 (154.9762, 186.4815) -> (154.8907, 186.6211) construction
  line L5155 (154.8907, 186.6211) -> (154.8059, 186.7614) construction
  line L5156 (154.8059, 186.7614) -> (154.7218, 186.9023) construction
  line L5157 (154.7218, 186.9023) -> (154.6383, 187.0438) construction
  line L5158 (154.6383, 187.0438) -> (154.5555, 187.186) construction
  line L5159 (154.5555, 187.186) -> (154.4733, 187.3288) construction
  line L5160 (154.4733, 187.3288) -> (154.3917, 187.4721) construction
  line L5161 (154.3917, 187.4721) -> (154.3108, 187.6161) construction
  line L5162 (154.3108, 187.6161) -> (154.2306, 187.7607) construction
  line L5163 (154.2306, 187.7607) -> (154.151, 187.9058) construction
  line L5164 (154.151, 187.9058) -> (154.072, 188.0515) construction
  line L5165 (154.072, 188.0515) -> (153.9937, 188.1978) construction
  line L5166 (153.9937, 188.1978) -> (153.916, 188.3447) construction
  line L5167 (153.916, 188.3447) -> (153.8389, 188.4921) construction
  line L5168 (153.8389, 188.4921) -> (153.7625, 188.6401) construction
  line L5169 (153.7625, 188.6401) -> (153.6867, 188.7886) construction
  line L5170 (153.6867, 188.7886) -> (153.6115, 188.9377) construction
  line L5171 (153.6115, 188.9377) -> (153.537, 189.0873) construction
  line L5172 (153.537, 189.0873) -> (153.463, 189.2374) construction
  line L5173 (153.463, 189.2374) -> (153.3897, 189.3881) construction
  line L5174 (153.3897, 189.3881) -> (153.3171, 189.5393) construction
  line L5175 (153.3171, 189.5393) -> (153.245, 189.6909) construction
  line L5176 (153.245, 189.6909) -> (153.1736, 189.8431) construction
  line L5177 (153.1736, 189.8431) -> (153.1169, 189.9653) construction
  line L5178 (153.1169, 189.9653) -> (153.0747, 190.0572) construction
  line L5179 (153.0747, 190.0572) -> (153.0467, 190.1185) construction
  line L5180 (153.0467, 190.1185) -> (153.0327, 190.1492) construction
  arc A137 (144.9129, 174.2132) -> (143.5184, 169.9215) centre (212.132, 150) ccw
  arc A138 (155.697, 160.6816) -> (154.1697, 163.005) centre (153.7319, 161.0535) ccw
  line L5181 (157.5954, 173.5481) -> (156.0975, 174.1948)
  line L5182 (157.5954, 126.4519) -> (156.0975, 125.8052)
  arc A139 (155.6851, 193.8) -> (153.0327, 190.1492) centre (212.132, 150) ccw
  arc A140 (161.7599, 177.5982) -> (160.1966, 174.5301) centre (212.132, 150) ccw
  arc A141 (143.5184, 130.0785) -> (144.9129, 125.7868) centre (212.132, 150) ccw
  arc A142 (157.5954, 173.5481) -> (160.1966, 174.5301) centre (158.3882, 175.3842) ccw
  spline S69 degree 5 poles (156.0975, 125.8052) (156.0692, 125.7929) (156.0122, 125.7692) (155.9258, 125.736) (155.8091, 125.6961) (155.6609, 125.6522) (155.5112, 125.6127) (155.3606, 125.5759) (155.2094, 125.5405) (155.0579, 125.506) (154.906, 125.4726) (154.7537, 125.4406) (154.6008, 125.4104) (154.4472, 125.3824) (154.2929, 125.3565) (154.138, 125.3326) (153.9826, 125.3103) (153.8268, 125.2895) (153.6706, 125.2699) (153.5141, 125.2515) (153.3573, 125.2342) (153.2002, 125.2182) (153.0427, 125.2035) (152.8849, 125.1902) (152.7267, 125.1782) (152.5682, 125.1675) (152.4094, 125.158) (152.2503, 125.1496) (152.0909, 125.1423) (151.9313, 125.1362) (151.7715, 125.1311) (151.6114, 125.1271) (151.4511, 125.1243) (151.2905, 125.1224) (151.1297, 125.1217) (150.9687, 125.122) (150.8075, 125.1234) (150.6461, 125.1258) (150.4845, 125.1292) (150.3227, 125.1335) (150.1608, 125.1389) (149.9986, 125.1452) (149.8363, 125.1525) (149.6739, 125.1608) (149.5113, 125.17) (149.3485, 125.1801) (149.1856, 125.1912) (149.0225, 125.2033) (148.8593, 125.2162) (148.696, 125.23) (148.5325, 125.2448) (148.3689, 125.2604) (148.2052, 125.277) (148.0414, 125.2944) (147.8775, 125.3127) (147.7135, 125.3319) (147.5494, 125.352) (147.3852, 125.3729) (147.2209, 125.3946) (147.0565, 125.4172) (146.892, 125.4407) (146.7274, 125.465) (146.5628, 125.4902) (146.398, 125.5161) (146.2333, 125.5429) (146.0684, 125.5706) (145.9035, 125.599) (145.7385, 125.6282) (145.5735, 125.6583) (145.4084, 125.6892) (145.2433, 125.7208) (145.1112, 125.7468) (145.0121, 125.7666) (144.946, 125.78) (144.9129, 125.7868) knots 0 0 0 0 0 0 0.01428571 0.02857143 0.04285714 0.05714286 0.07142857 0.08571429 0.1 0.11428571 0.12857143 0.14285714 0.15714286 0.17142857 0.18571429 0.2 0.21428571 0.22857143 0.24285714 0.25714286 0.27142857 0.28571429 0.3 0.31428571 0.32857143 0.34285714 0.35714286 0.37142857 0.38571429 0.4 0.41428571 0.42857143 0.44285714 0.45714286 0.47142857 0.48571429 0.5 0.51428571 0.52857143 0.54285714 0.55714286 0.57142857 0.58571429 0.6 0.61428571 0.62857143 0.64285714 0.65714286 0.67142857 0.68571429 0.7 0.71428571 0.72857143 0.74285714 0.75714286 0.77142857 0.78571429 0.8 0.81428571 0.82857143 0.84285714 0.85714286 0.87142857 0.88571429 0.9 0.91428571 0.92857143 0.94285714 0.95714286 0.97142857 0.98571429 1 1 1 1 1 1
  line L5183 (156.0975, 125.8052) -> (156.0692, 125.7929) construction
  line L5184 (156.0692, 125.7929) -> (156.0122, 125.7692) construction
  line L5185 (156.0122, 125.7692) -> (155.9258, 125.736) construction
  line L5186 (155.9258, 125.736) -> (155.8091, 125.6961) construction
  line L5187 (155.8091, 125.6961) -> (155.6609, 125.6522) construction
  line L5188 (155.6609, 125.6522) -> (155.5112, 125.6127) construction
  line L5189 (155.5112, 125.6127) -> (155.3606, 125.5759) construction
  line L5190 (155.3606, 125.5759) -> (155.2094, 125.5405) construction
  line L5191 (155.2094, 125.5405) -> (155.0579, 125.506) construction
  line L5192 (155.0579, 125.506) -> (154.906, 125.4726) construction
  line L5193 (154.906, 125.4726) -> (154.7537, 125.4406) construction
  line L5194 (154.7537, 125.4406) -> (154.6008, 125.4104) construction
  line L5195 (154.6008, 125.4104) -> (154.4472, 125.3824) construction
  line L5196 (154.4472, 125.3824) -> (154.2929, 125.3565) construction
  line L5197 (154.2929, 125.3565) -> (154.138, 125.3326) construction
  line L5198 (154.138, 125.3326) -> (153.9826, 125.3103) construction
  line L5199 (153.9826, 125.3103) -> (153.8268, 125.2895) construction
  line L5200 (153.8268, 125.2895) -> (153.6706, 125.2699) construction
  line L5201 (153.6706, 125.2699) -> (153.5141, 125.2515) construction
  line L5202 (153.5141, 125.2515) -> (153.3573, 125.2342) construction
  line L5203 (153.3573, 125.2342) -> (153.2002, 125.2182) construction
  line L5204 (153.2002, 125.2182) -> (153.0427, 125.2035) construction
  line L5205 (153.0427, 125.2035) -> (152.8849, 125.1902) construction
  line L5206 (152.8849, 125.1902) -> (152.7267, 125.1782) construction
  line L5207 (152.7267, 125.1782) -> (152.5682, 125.1675) construction
  line L5208 (152.5682, 125.1675) -> (152.4094, 125.158) construction
  line L5209 (152.4094, 125.158) -> (152.2503, 125.1496) construction
  line L5210 (152.2503, 125.1496) -> (152.0909, 125.1423) construction
  line L5211 (152.0909, 125.1423) -> (151.9313, 125.1362) construction
  line L5212 (151.9313, 125.1362) -> (151.7715, 125.1311) construction
  line L5213 (151.7715, 125.1311) -> (151.6114, 125.1271) construction
  line L5214 (151.6114, 125.1271) -> (151.4511, 125.1243) construction
  line L5215 (151.4511, 125.1243) -> (151.2905, 125.1224) construction
  line L5216 (151.2905, 125.1224) -> (151.1297, 125.1217) construction
  line L5217 (151.1297, 125.1217) -> (150.9687, 125.122) construction
  line L5218 (150.9687, 125.122) -> (150.8075, 125.1234) construction
  line L5219 (150.8075, 125.1234) -> (150.6461, 125.1258) construction
  line L5220 (150.6461, 125.1258) -> (150.4845, 125.1292) construction
  line L5221 (150.4845, 125.1292) -> (150.3227, 125.1335) construction
  line L5222 (150.3227, 125.1335) -> (150.1608, 125.1389) construction
  line L5223 (150.1608, 125.1389) -> (149.9986, 125.1452) construction
  line L5224 (149.9986, 125.1452) -> (149.8363, 125.1525) construction
  line L5225 (149.8363, 125.1525) -> (149.6739, 125.1608) construction
  line L5226 (149.6739, 125.1608) -> (149.5113, 125.17) construction
  line L5227 (149.5113, 125.17) -> (149.3485, 125.1801) construction
  line L5228 (149.3485, 125.1801) -> (149.1856, 125.1912) construction
  line L5229 (149.1856, 125.1912) -> (149.0225, 125.2033) construction
  line L5230 (149.0225, 125.2033) -> (148.8593, 125.2162) construction
  line L5231 (148.8593, 125.2162) -> (148.696, 125.23) construction
  line L5232 (148.696, 125.23) -> (148.5325, 125.2448) construction
  line L5233 (148.5325, 125.2448) -> (148.3689, 125.2604) construction
  line L5234 (148.3689, 125.2604) -> (148.2052, 125.277) construction
  line L5235 (148.2052, 125.277) -> (148.0414, 125.2944) construction
  line L5236 (148.0414, 125.2944) -> (147.8775, 125.3127) construction
  line L5237 (147.8775, 125.3127) -> (147.7135, 125.3319) construction
  line L5238 (147.7135, 125.3319) -> (147.5494, 125.352) construction
  line L5239 (147.5494, 125.352) -> (147.3852, 125.3729) construction
  line L5240 (147.3852, 125.3729) -> (147.2209, 125.3946) construction
  line L5241 (147.2209, 125.3946) -> (147.0565, 125.4172) construction
  line L5242 (147.0565, 125.4172) -> (146.892, 125.4407) construction
  line L5243 (146.892, 125.4407) -> (146.7274, 125.465) construction
  line L5244 (146.7274, 125.465) -> (146.5628, 125.4902) construction
  line L5245 (146.5628, 125.4902) -> (146.398, 125.5161) construction
  line L5246 (146.398, 125.5161) -> (146.2333, 125.5429) construction
  line L5247 (146.2333, 125.5429) -> (146.0684, 125.5706) construction
  line L5248 (146.0684, 125.5706) -> (145.9035, 125.599) construction
  line L5249 (145.9035, 125.599) -> (145.7385, 125.6282) construction
  line L5250 (145.7385, 125.6282) -> (145.5735, 125.6583) construction
  line L5251 (145.5735, 125.6583) -> (145.4084, 125.6892) construction
  line L5252 (145.4084, 125.6892) -> (145.2433, 125.7208) construction
  line L5253 (145.2433, 125.7208) -> (145.1112, 125.7468) construction
  line L5254 (145.1112, 125.7468) -> (145.0121, 125.7666) construction
  line L5255 (145.0121, 125.7666) -> (144.946, 125.78) construction
  line L5256 (144.946, 125.78) -> (144.9129, 125.7868) construction
  arc A143 (153.0327, 109.8508) -> (155.6851, 106.2) centre (212.132, 150) ccw